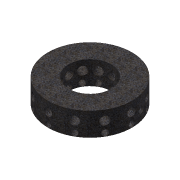
# Autodesk Inventor part: 2h4cem
Saved by Autodesk Inventor 2017 (Build 210142000, 142)
## iProperties
Company: HERA Project
Created: 2013-05-20
Part Number: 2h4cem
Material: Concrete
Document SubType Name: Modeling
Designer: David DeBoer
Density: 2.40731 g/cm^3
Description: Hub cement
Mass: 233879 g
Surface Area: 30868 cm^2
Volume: 97153.7 cm^3
Appearance: Exposed Aggregate - Coarse
Author: David DeBoer
Title: Cement
Autodesk Inventor part; units mm, degrees
ref_plane "YZ Plane" through (0, 0, 0) normal (1, 0, 0) x (0, 1, 0)
ref_plane "XZ Plane" through (0, 0, 0) normal (0, 1, 0) x (-1, 0, 0)
ref_plane "XY Plane" through (0, 0, 0) normal (0, 0, 1) x (1, 0, 0)
sketch "Sketch1" plane through (0, 0, 0) normal (0, 1, 0) x (-1, 0, 0)
  circle A0 centre (1.7415, 0) radius 455.93
  circle A1 centre (1.7415, 0) radius 231.14
  point P0 (0, 0)
  dimension "d0" = 911.86
  dimension "d4" = 462.28
  constraints: 2 centre point
  measures "d0" diameter of A0
  measures "d4" diameter of A1
extrude "Extrusion1" add sketch "Sketch1" along normal blind 254
sketch "Sketch2" plane through (-1.7415, 254, 0) normal (0, 1, 0) x (1, 0, 0)
  circle A0 centre (0, 0) radius 231.14 projected
  circle A1 centre (0, 0) radius 455.93 projected
  point P0 (1.7415, 0)
  point P1 (455.93, 0)
  constraints: 1 horizontal alignment, 1 other
ref_plane "Work Plane1" through (454.1885, 254, 0) normal (1, 0, 0) x (0, 1, 0)
sketch "Sketch5" plane through (-1.7415, 254, 0) normal (0, 1, 0) x (1, 0, 0)
  circle A0 centre (0, 0) radius 231.14 projected
  circle A1 centre (0, 0) radius 455.93 projected
  point P0 (1.7415, 0)
  point P1 (1.7611, 455.9266)
  constraints: 2 other
ref_plane "Work Plane2" through (0.0196, 254, -455.9266) normal (0.0038627, 0, -0.9999925) x (-0.9999925, 0, -0.0038627)
sketch "Sketch6" plane through (0.0196, 254, -455.9266) normal (0.0038627, 0, -0.9999925) x (-0.9999925, 0, -0.0038627)
  circle A0 centre (-1.7415, -104) radius 45.5
  line L0 (-455.93, -254) -> (455.93, -254) projected
  circle A1 centre (0, -218.5) radius 32
  point P0 (-1.7415, -254)
  dimension "d15" = 91
  dimension "d17" = 150
  dimension "d18" = 64
  dimension "d19" = 35.5
  constraints: 2 centre point
  measures "d15" diameter of A0
  measures "d17" distance from line of A0.centre L0
  measures "d18" diameter of A1
  measures "d19" distance from line of L0 A1.centre
extrude "Extrusion4" cut sketch "Sketch6" against normal blind 254
pattern_circular "Circular Pattern1" count 12 over 360 about axis through (-1.7415, 0, 0) along (0, 1, 0) of "Extrusion4"
sketch "Sketch7" plane through (-1.7415, 254, 0) normal (0, 1, 0) x (1, 0, 0)
  circle A0 centre (0, 0) radius 231.14 projected
  circle A1 centre (0, 0) radius 455.93 projected
  line L0 (1.7415, 0) -> (492.4318, 131.4801) construction
  line L1 (1.7415, 0) -> (509.7415, 0) construction
  point P0 (440.511, 117.5679)
  dimension "d25" = 508
  dimension "d26" = 15
  constraints: 4 end point, 1 horizontal, 1 point on line, 2 other
  measures "d25" distance of L0.start L0.end
  measures "d26" angle of L1 L0
ref_plane "Work Plane3" through (438.7695, 254, -117.5679) normal (0.9661812, 0, -0.257864) x (0, 1, 0)
sketch "Sketch8" plane through (438.7695, 254, -117.5679) normal (0.9661812, 0, -0.257864) x (0, 1, 0)
  circle A0 centre (-152.4, 0.4491) radius 30.1625
  line L0 (-254, 455.93) -> (-254, -455.93) projected
  point P0 (-254, 0.4491)
  dimension "d27" = 60.325
  dimension "d28" = 101.6
  constraints: 1 centre point
  measures "d27" diameter of A0
  measures "d28" distance from line of A0.centre L0
extrude "Extrusion5" cut sketch "Sketch8" against normal blind 254
sketch "Sketch9" plane through (-1.7415, 0, 0) normal (0, -1, 0) x (1, 0, 0)
  line L0 (0, 0) -> (322.3912, 322.3912) construction
  circle A0 centre (0, 0) radius 455.93 projected
  line L1 (0, 0) -> (455.93, 0) construction
  line L2 (0, 0) -> (118.0034, -440.3946) construction
  line L3 (0, 0) -> (-440.3946, 118.0034) construction
  circle A1 centre (-368.0177, 98.6101) radius 5
  circle A2 centre (269.4077, 269.4077) radius 5
  circle A3 centre (98.6101, -368.0177) radius 5
  dimension "d35" = 45
  dimension "d36" = 120
  dimension "d37" = 120
  dimension "d38" = 10
  dimension "d39" = 10
  dimension "d40" = 10
  dimension "d41" = 381
  dimension "d42" = 381
  dimension "d43" = 381
  constraints: 8 end point, 3 centre point, 3 point on circle, 3 point on line, 1 equal length, 1 horizontal
  measures "d35" angle of L1 L0
  measures "d36" angle of L2 L0
  measures "d37" angle of L3 L2
  measures "d38" diameter of A1
  measures "d39" diameter of A2
  measures "d40" diameter of A3
  measures "d41" distance of L0.start A3.centre
  measures "d42" distance of A2.centre L0.start
  measures "d43" distance of A1.centre L0.start
extrude "Extrusion6" cut sketch "Sketch9" against normal blind 203.2 contours A1 | A2 | A3
body "Solid1"
